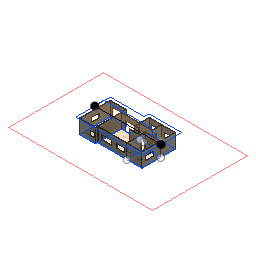
Day13 - House plans (Autodesk Fusion 360 design; units mm, degrees)
Autodesk Fusion 360 part; units mm, degrees
sketch "Sketch1" plane through (0, 0, 0) normal (0, 0, 1) x (1, 0, 0)
  line L0 (-2990.1281, -3865.3597) -> (-6454.0292, -3865.3597)
  line L1 (-6454.0292, -3865.3597) -> (-6454.0292, 2708.9832)
  line L2 (-6454.0292, 2708.9832) -> (-2990.1281, 2708.9832)
  line L3 (-2990.1281, 2708.9832) -> (-2990.1281, -3865.3597)
  line L4 (-2990.1281, -3427.0701) -> (6369.4739, -3427.0701)
  line L5 (6369.4739, -3427.0701) -> (6369.4739, 3698.6692)
  line L6 (6369.4739, 3698.6692) -> (809.4029, 3698.6692)
  line L7 (-2990.1281, 2708.9832) -> (-2990.1281, -3427.0701)
  line L8 (-2990.1281, 1685.2306) -> (809.4029, 1685.2306)
  line L9 (809.4029, 1685.2306) -> (809.4029, 3698.6692)
  line L10 (-2990.1281, 2708.9832) -> (-2990.1281, 1685.2306)
  line L11 (6369.4739, 599.0251) -> (3100.141, 599.0251)
  line L12 (3100.141, 599.0251) -> (3100.141, -3427.0701)
  line L13 (3100.141, -3427.0701) -> (6369.4739, -3427.0701)
  line L14 (6369.4739, -3427.0701) -> (6369.4739, 599.0251)
  line L15 (3100.141, -570.2441) -> (786.5447, -570.2441)
  line L16 (786.5447, -570.2441) -> (786.5447, -470.2441)
  line L17 (786.5447, -470.2441) -> (3100.141, -470.2441)
  line L18 (3100.141, -470.2441) -> (3100.141, -570.2441)
  line L19 (-3090.1281, -3765.3597) -> (-6354.0292, -3765.3597)
  line L20 (-6354.0292, -3765.3597) -> (-6354.0292, 2608.9832)
  line L21 (-6354.0292, 2608.9832) -> (-3090.1281, 2608.9832)
  line L22 (-3090.1281, 2608.9832) -> (-3090.1281, -3765.3597)
  line L23 (-2890.1281, -3327.0701) -> (6269.4739, -3327.0701)
  line L24 (6269.4739, -3327.0701) -> (6269.4739, 3598.6692)
  line L25 (6269.4739, 3598.6692) -> (909.4029, 3598.6692)
  line L26 (909.4029, 1585.2306) -> (909.4029, 3598.6692)
  line L27 (-2890.1281, 1585.2306) -> (909.4029, 1585.2306)
  line L28 (-2890.1281, -3327.0701) -> (-2990.1281, -3329.4228)
  line L29 (-2890.1281, 1585.2306) -> (-2990.1281, 1585.2306)
  line L30 (6369.4739, 499.0251) -> (3200.141, 499.0251)
  line L31 (3200.141, 499.0251) -> (3200.141, -3427.0701)
  line L32 (809.4029, 1585.2306) -> (3521.6455, 1585.2306)
  line L33 (3521.6455, 1585.2306) -> (3521.6455, 3698.6692)
  line L34 (3521.6455, 3698.6692) -> (809.4029, 3698.6692)
  line L35 (809.4029, 3698.6692) -> (809.4029, 1585.2306)
  line L36 (809.4029, 1685.2306) -> (3421.6455, 1685.2306)
  line L37 (3421.6455, 1685.2306) -> (3421.6455, 3698.6692)
  line L38 (809.4029, 1585.2306) -> (809.4029, 505.694)
  line L39 (809.4029, 505.694) -> (1648.7831, 505.694)
  line L40 (1648.7831, 505.694) -> (1648.7831, 700.6388)
  line L41 (909.4029, 1585.2306) -> (909.4029, 605.694)
  line L42 (909.4029, 605.694) -> (1548.7831, 605.694)
  line L43 (1548.7831, 605.694) -> (1548.7831, 700.6388)
  line L44 (1548.7831, 700.6388) -> (1648.7831, 700.6388)
  line L45 (1294.9886, 3698.6692) -> (1294.9886, 3598.6692)
  line L46 (2111.9261, 3698.6692) -> (2111.9261, 3598.6692)
  line L47 (4048.6551, 3698.6692) -> (4048.6551, 3598.6692)
  line L48 (5700.4654, 3698.6692) -> (5700.4654, 3598.6692)
  line L49 (3421.6455, 2516.11) -> (3521.6455, 2516.11)
  line L50 (3421.6455, 1752.6279) -> (3521.6455, 1752.6279)
  line L51 (2545.6999, 1685.2306) -> (2545.6999, 1585.2306)
  line L52 (1714.993, 1685.2306) -> (1714.993, 1585.2306)
  line L53 (3100.141, 441.8435) -> (3200.141, 499.0251)
  line L54 (3100.141, -380.6989) -> (3200.141, -380.6989)
  line L55 (6269.4739, -943.1211) -> (6369.4739, -943.1211)
  line L56 (6269.4739, -2581.1757) -> (6369.4739, -2581.1757)
  line L57 (-2141.6835, 1685.2306) -> (-2141.6835, 1585.2306)
  line L58 (-94.0993, 1685.2306) -> (-94.0993, 1585.2306)
  line L59 (-5907.6305, 2708.9832) -> (-5907.6305, 2608.9832)
  line L60 (-3430.4296, 2708.9832) -> (-3430.4296, 2608.9832)
  line L61 (-6454.0292, 253.7511) -> (-6354.0292, 253.7511)
  line L62 (-6454.0292, -1382.2244) -> (-6354.0292, -1382.2244)
  line L63 (-4063.1748, -3765.3597) -> (-4063.1748, -3865.3597)
  line L64 (-3190.1129, -3765.3597) -> (-3190.1129, -3865.3597)
  line L65 (-3090.1281, -3226.6773) -> (-2990.1281, -3219.9614)
  line L66 (-3090.1281, -2360.3312) -> (-2990.1281, -2367.047)
  line L67 (-2169.3019, -3327.0701) -> (-2169.3019, -3427.0701)
  line L68 (-94.1008, -3327.0701) -> (-94.1008, -3427.0701)
  line L69 (1086.3361, -3327.0701) -> (1086.3361, -3427.0701)
  line L70 (2750.0365, -3327.0701) -> (2750.0365, -3427.0701)
  dimension "d1" = 100
  dimension "d3" = 100
  dimension "d4" = -100
  dimension "d5" = -100
  dimension "d6" = -100
  measures "d1" distance of L0
  measures "d4" distance of L11
  measures "d5" distance of L32
  measures "d6" distance of L38
extrude "Extrude1" add sketch "Sketch1" along normal blind 3000 contours L0 L3 L7 L19 L22 L64 L65 | L0 L19 L63 L64 | L3 L4 L7 L23 L28 L67 | L0 L1 L19 L20 L62 L63 | L4 L23 L67 L68 | L4 L23 L68 L69 | L1 L20 L61 L62 | L2 L3 L7 L10 L21 L22 L60 L66 | L4 L23 L69 L70 | L1 L2 L20 L21 L59 L61 | L3 L7 L8 L27 L29 L57 | L4 L12 L23 L70 | L4 L12 L13 L23 L31 | L4 L5 L13 L14 L23 L24 L31 L56 | L12 L18 L23 L31 L54 | L8 L27 L35 L58 | L12 L15 L16 L17 L18 | L26 L27 L32 L35 L36 | L6 L9 L25 L26 L34 L35 L36 L45 | L27 L32 L38 L39 L40 L41 L42 L43 L44 | L5 L14 L24 L55 L56 | L26 L32 L36 L52 | L5 L14 L24 L30 L55 | L11 L12 L24 L30 L53 | L6 L25 L34 L45 L46 | L5 L11 L14 L24 L30 | L6 L25 L34 L37 L46 | L32 L33 L36 L37 L50 L51 | L5 L6 L11 L24 L25 L48 | L6 L25 L33 L34 L37 | L6 L25 L33 L47 | L25 L33 L37 L49 | L6 L25 L47 L48 makes body 1 at (129.7392, -3427.0701, 1000) makes body 2 at (2871.0151, 1585.2306, 1000) makes body 3 at (-3090.1281, 952.545, 1000)
extrude "Extrude2" cut sketch "Sketch1" along normal blind 900 from surface at 1000 contours L0 L19 L63 L64 | L4 L23 L67 L68 | L1 L20 L61 L62 | L4 L23 L69 L70 | L5 L14 L24 L55 L56 | L6 L25 L34 L45 L46 | L6 L25 L47 L48 bodies 1
extrude "Extrude3" add sketch "Sketch1" along normal blind 1000 from surface at 2000 contours L3 L7 L22 L65 L66 | L2 L21 L59 L60 | L8 L27 L57 L58 | L12 L31 L53 L54 | L32 L36 L51 L52 | L33 L37 L49 L50 bodies 1 2 3
sketch "Sketch2" plane through (0, 0, 3000) normal (0, 0, 1) x (-1, 0, 0)
  line L0 (7020.2567, -3282.1442) -> (-157.9932, -3282.1442)
  line L1 (-157.9932, -3282.1442) -> (-157.9932, -4307.6085)
  line L2 (-157.9932, -4307.6085) -> (-6983.7398, -4307.6085)
  line L3 (-6983.7398, -4307.6085) -> (-6983.7398, 4040.3116)
  line L4 (-6983.7398, 4040.3116) -> (7004.2338, 4040.3116)
  line L5 (7004.2338, 4040.3116) -> (7020.2567, -3282.1442)
sketch "Sketch3" plane through (0, 0, 0) normal (0, 1, 0) x (1, 0, 0)
  line L0 (6983.7398, -3000) -> (4583.9009, -4982.1418)
  line L1 (4583.9009, -4982.1418) -> (-5175.4891, -4982.1418)
  line L2 (-5175.4891, -4982.1418) -> (-7004.2338, -3000)
  line L3 (-7004.2338, -3000) -> (6983.7398, -3000)
